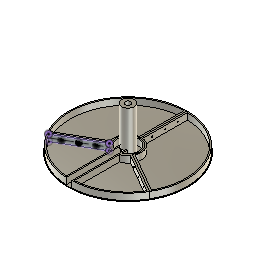
Base For Lamp (Autodesk Fusion 360 design; units mm, degrees)
Autodesk Fusion 360 part; units mm, degrees
note: some values were not read from the file. Chosen so that the rebuilt part matches the saved one: which face or edge a step refers to. Set by a fixed rule: which sketch regions a step uses.
sketch "Base" plane through (0, 0, 0) normal (0, 0, 1) x (1, 0, 0)
  circle A0 centre (0, 0) radius 140
  circle A1 centre (0, 0) radius 138.5
  circle A2 centre (0, 0) radius 135.5
  circle A3 centre (0, 0) radius 6.5
  circle A4 centre (0, 0) radius 12.5
  circle A5 centre (0, 0) radius 14.5
  line L0 (0, 0) -> (0, -66.8825) construction
  line L1 (6.5, -12.9615) -> (6.5, -138.3474)
  line L2 (-6.5, -12.9615) -> (-6.5, -138.3474)
  dimension "d4" = 280
  dimension "d5" = 277
  dimension "d6" = 3
  dimension "d7" = 13
  dimension "d8" = 25
  dimension "d14" = 2
  dimension "d20" = 13
  constraint coincident A0.centre A1.centre
  constraint concentric A0 A2
  constraint concentric A3 A5
  constraint vertical L0
  constraint coincident A5 L1.start
  constraint coincident A1 L1.end
  constraint vertical L1
  constraint symmetric L0 L1.start L2.start
  constraint symmetric L0 L1.end L2.end
  measures "d4" diameter of A0
  measures "d5" diameter of A1
  measures "d6" distance of A1 A2
  measures "d7" diameter of A3
  measures "d8" diameter of A4
  measures "d14" distance of A4 A5
  measures "d20" distance of L1 L2
extrude "Extrude1" add sketch "Base" along normal blind 15 contours A1 A2 L1 L2 | A1 A2 L1 L2 makes body 1
extrude "Extrude2" add sketch "Base" against normal blind 1 contours A0 | A1 A2 L1 L2 | A1 A2 L1 L2 | A2 A5 L1 L2 | A2 A5 L1 L2 | A5 bodies 1
extrude "Extrude3" add sketch "Base" along normal blind 100 contours A5 | A4 bodies 1
extrude "Extrude4" cut sketch "Base" along normal blind 20 contours A4 bodies 1
chamfer "Chamfer1" distance 1 angle 45 1 edges at (-11.6541, -4.5202, 20) on bodies 1
extrude "Extrude5" cut sketch "Base" along normal blind 15 contours A1 A2 L1 L2 picked at (-5.0558, -136.3914) bodies 1
ref_plane "WorkPlane1" through (-6.5, -138.3474, 0) normal (0, -1, 0) x (1, 0, 0)
sketch "Hole in center" plane through (0, -138.3474, 0) normal (0, -1, 0) x (-1, 0, 0)
  line L0 (0, 0) -> (0, -12.9368) construction
  line L1 (6.5, 0) -> (6.5, -15)
  line L2 (0, -12.9368) -> (3, -12.9368)
  line L3 (3, -12.9368) -> (6.5, -10)
  line L4 (-3, -12.9368) -> (-6.5, -10)
  line L5 (0, -12.9368) -> (-3, -12.9368)
  line L6 (-140, 0) -> (140, 0)
  line L7 (-138.5, 0) -> (138.5, 0)
  line L8 (-6.5, -15) -> (-6.5, 0)
  dimension "d23" = 50
  dimension "d24" = 6
  dimension "d25" = 10
  constraint coincident L0.start origin
  constraint vertical L0
  constraint perpendicular L0 L2
  constraint coincident L1 L3.end
  constraint symmetric L2.start L0 L5.start
  constraint symmetric L0 L2.end L4.start
  constraint symmetric L0 L3.end L4.end
  measures "d23" angle of L1 L3
  measures "d24" distance of L2.end L4.start
  measures "d25" distance of L4.end L6
sketch "Trough for wire" plane through (0, 0, 0) normal (0, 0, 1) x (-1, 0, 0)
  circle A0 centre (0, 0) radius 140
  circle A1 centre (0, 0) radius 14.5
  arc A2 (-6.5, 135.344) -> (6.5, 135.344) centre (0, 0) ccw
  line L0 (6.5, 135.344) -> (6.5, 138.3474)
  arc A3 (-6.5, 138.3474) -> (6.5, 138.3474) centre (0, 0) ccw
  line L1 (-6.5, 138.3474) -> (-6.5, 135.344)
  line L2 (-6.5, 135.344) -> (-6.5, 12.9615)
  line L3 (-9.5, 135.1666) -> (-9.5, 10.9545)
  line L4 (0, -2.5) -> (0, -20)
  line L5 (9.5, 135.1666) -> (9.5, 10.9545)
  line L6 (6.5, 135.344) -> (6.5, 12.9615)
  dimension "d32" = 3
  constraint coincident A2.start L1.end
  constraint coincident A1 L2.end
  constraint parallel L1 L2
  constraint coincident A2 L3.start
  constraint coincident A1 L3.end
  constraint vertical L3
  constraint symmetric A2.start L4 A2.end
  constraint symmetric L2.end L4 L6.end
  constraint symmetric L3.start L4 L5.start
  constraint symmetric L3.end L4 L5.end
  measures "d32" distance of L2 L3
extrude "Extrude8" add sketch "Trough for wire" along normal blind 15 contours A1 A2 L5 L6 | A1 A2 L2 L3 bodies 1
sketch "Make 3d printable" plane through (0, 0, 0) normal (0, 0, 1) x (-1, 0, 0)
  line L0 (9.5, 135.1666) -> (9.5, 10.9545)
  arc A0 (-9.5, 10.9545) -> (9.5, 10.9545) centre (0, 0) ccw
  line L1 (-9.5, 10.9545) -> (-9.5, 135.1666)
  arc A1 (-9.5, 135.1666) -> (9.5, 135.1666) centre (0, 0) ccw
  circle A2 centre (0, 0) radius 25
  line L2 (-9.5, 135.1666) -> (-9.5, 10.9545)
  circle A3 centre (0, 0) radius 140
  line L3 (0, -140) -> (0, -28)
  arc A4 (-9.5, 135.1666) -> (9.5, 135.1666) centre (0, 0) ccw
  line L4 (-4, -135.4409) -> (-4, -27.7128)
  line L5 (4, -135.4409) -> (4, -27.7128)
  line L6 (115.2953, 71.1846) -> (22, 17.3205)
  line L7 (121.2436, 70) -> (24.2487, 14)
  line L8 (119.2953, 64.2564) -> (26, 10.3923)
  line L9 (-119.2953, 64.2564) -> (-26, 10.3923)
  line L10 (-121.2436, 70) -> (-24.2487, 14)
  line L11 (-115.2953, 71.1846) -> (-22, 17.3205)
  arc A5 (-28.6224, 11.9063) -> (-4, -30.7409) centre (0, 0) ccw
  arc A6 (4, -30.7409) -> (28.6224, 11.9063) centre (0, 0) ccw
  arc A7 (24.6224, 18.8345) -> (9.5, 29.5085) centre (0, 0) ccw
  arc A8 (-9.5, 10.1036) -> (-11.4386, 7.8417) centre (0, 0) ccw
  arc A9 (-9.5, 29.5085) -> (-24.6224, 18.8345) centre (0, 0) ccw
  arc A10 (-24.2487, 14) -> (24.2487, 14) centre (0, 0) ccw
  arc A11 (-22, 17.3205) -> (-24.2487, 14) centre (0, 0) ccw
  arc A12 (24.2487, 14) -> (22, 17.3205) centre (0, 0) ccw
  dimension "d35" = 50
  dimension "d36" = 3
  dimension "d37" = 4
  dimension "d39" = 360
  dimension "d40" = 3
  dimension "d41" = 3
  dimension "d42" = 3
  dimension "d43" = 3
  constraint coincident A0.centre A1.centre
  constraint concentric A2 A10
  constraint coincident A3 L3.start
  constraint coincident L3.end A10
  constraint vertical L3
  constraint coincident L3 A0.centre
  constraint coincident A4 L4.start
  constraint coincident L4.end A10
  constraint vertical L4
  constraint symmetric L3 L4.start L5.start
  constraint symmetric L3 L4.end L5.end
  constraint coincident L9 A5.start
  constraint coincident L4 A5.end
  constraint coincident L5 A6.start
  constraint coincident L8 A6.end
  constraint coincident L0 A7.end
  constraint coincident L6 A7.start
  constraint coincident L11 A8.start
  constraint coincident L1 A8.start
  constraint coincident L2 A9.start
  constraint coincident L11 A9.end
  constraint concentric A10 A11
  constraint concentric A10 A12
  measures "d35" diameter of A2
  measures "d36" distance of A2 A10
  measures "d37" distance of L3 L4
  measures "d40" distance of A5 A10
  measures "d41" distance of A6 A10
  measures "d42" distance of A7 A10
  measures "d43" distance of A9 A10
extrude "Extrude9" add sketch "Make 3d printable" along normal blind 15 contours L0 L1 A2 L2 L6 L11 A7 A9 A10 A11 A12 | A1 A4 L6 L7 A12 | A1 A4 L7 L8 A10 | A1 L3 A4 L5 A10 | L5 L8 A6 A10 | A1 A4 L10 L11 A11 | A1 L3 A4 L4 A10 | A1 A4 L9 L10 A10 | L4 L9 A5 A10 bodies 1
sketch "Holes for bolting together" plane through (2, -3.4641, 0) normal (0.5, -0.866025, 0) x (0.866025, 0.5, 0)
  line L0 (-135.4409, 0) -> (-30.7409, 0)
  line L1 (-30.7409, 0) -> (-30.7409, 15)
  line L2 (-30.7409, 15) -> (-135.4409, 15)
  line L3 (-135.4409, 15) -> (-135.4409, 0)
  line L4 (-135.4409, 15) -> (-30.7409, 15)
  line L5 (-30.7409, 0) -> (-135.4409, 0)
  line L6 (-135.4409, 0) -> (-135.4409, 15)
  line L7 (-30.7409, 0) -> (-30.7409, 15)
  line L8 (-135.4409, 7.5) -> (-30.7409, 7.5) construction
  circle A0 centre (-83.0909, 7.5) radius 1.5
  circle A1 centre (-113.0909, 7.5) radius 1.5
  circle A2 centre (-53.0909, 7.5) radius 1.5
  dimension "d54" = 3
  dimension "d57" = 30
  dimension "d58" = 0
  constraint midpoint L6 L8.start
  constraint midpoint L1 L8.end
  constraint coincident L8 A0.centre
  constraint midpoint L8 A0.centre
  measures "d54" diameter of A0
extrude "Extrude16" cut sketch "Holes for bolting together" against normal blind 8 contours A0 | A1 | A2 bodies 1
pattern_circular "C-Pattern4" count 3 over 360 about axis through (0, 0, 1.75) along (0, 0, 1) of "Extrude16"
split "Split1" by curves path "Make 3d printable" along L7 A10 L10 bodies 1 makes body 2 at (102.1399, 7.5147, -1)
split "Split2" by curves path "Make 3d printable" along L3 bodies 2 makes body 3 at (-91.9382, -45.0492, -1)
extrude "Extrude13" cut sketch "Hole in center" against normal blind 138.347 bodies 1
sketch "Breakaway Support material " plane through (0, 0, -1) normal (0, 0, -1) x (1, 0, 0)
  line L0 (0, -140) -> (0, -28)
  arc A0 (-24.2487, 14) -> (0, -28) centre (0, 0) ccw
  line L1 (-24.2487, 14) -> (-121.2436, 70)
  arc A1 (-121.2436, 70) -> (0, -140) centre (0, 0) ccw
  circle A2 centre (0, 0) radius 6.5
  circle A3 centre (0, 0) radius 6.9
  dimension "d76" = 0.4
  constraint coincident A0.centre A1.centre
  measures "d76" distance of A2 A3
extrude "Extrude17" add sketch "Breakaway Support material " against normal blind 21 contours A3 bodies 1
equation "d40 = d36"
equation "d41 = d40"
equation "d42 = d40"
equation "d43 = d40"
named bodies: "Part1", "Part 2", "Part3"
